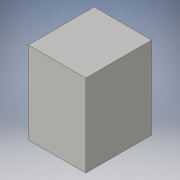
# Autodesk Inventor part: SwitchBlock
Saved by Autodesk Inventor 2016 (Build 200138000, 138)
## iProperties
Created: 2016-08-31
Part Number: SwitchBlock
Material: Generic
Document SubType Name: Modeling
Designer: jfixelle
Density: 1 g/cm^3
Appearance: Default
Author: jfixelle
Autodesk Inventor part; units mm, degrees
ref_plane "YZ Plane" through (0, 0, 0) normal (1, 0, 0) x (0, 1, 0)
ref_plane "XZ Plane" through (0, 0, 0) normal (0, 1, 0) x (-1, 0, 0)
ref_plane "XY Plane" through (0, 0, 0) normal (0, 0, 1) x (1, 0, 0)
sketch "Sketch1" plane through (0, 0, 0) normal (0, 1, 0) x (-1, 0, 0)
  line L0 (1.4826, 3.5355) -> (-5.5024, 3.5355)
  line L1 (-5.5024, 3.5355) -> (-5.5024, -4.4655)
  line L2 (-5.5024, -4.4655) -> (1.4826, -4.4655)
  line L3 (1.4826, -4.4655) -> (1.4826, 3.5355)
  point P0 (0, 0)
  dimension "d0" = 8.001
  dimension "d1" = 6.985
  constraints: 8 end point, 2 parallel, 1 horizontal, 1 perpendicular
  measures "d0" distance of L2.end L0.start
  measures "d1" distance of L1.end L2.end
extrude "Extrusion1" add sketch "Sketch1" along normal blind 10
body "Solid1"
